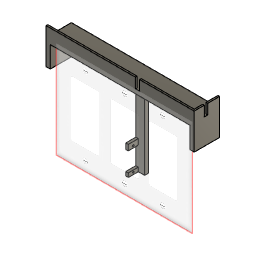
CPS_Project_Switch Mount v4 (Autodesk Fusion 360 design; units mm, degrees)
Autodesk Fusion 360 part; units mm, degrees
sketch "Sketch2" plane through (0, 0, 0) normal (0, 1, 0) x (1, 0, 0)
  line L0 (0, -62.2369) -> (87.5, -62.2369)
  line L1 (87.5, -62.2369) -> (87.5, -32.2369)
  line L2 (87.5, -32.2369) -> (82.5, -32.2369)
  line L3 (0, -57.2369) -> (0, -62.2369)
  line L4 (82.5, -32.2369) -> (82.5, -57.2369)
  line L5 (82.5, -57.2369) -> (0, -57.2369)
  line L6 (0, 0) -> (0, -57.2369) construction
  line L7 (-87.5, -32.2369) -> (-82.5, -32.2369)
  line L8 (-82.5, -32.2369) -> (-82.5, -57.2369)
  line L9 (-82.5, -57.2369) -> (0, -57.2369)
  line L10 (0, -57.2369) -> (0, -62.2369)
  line L11 (0, -62.2369) -> (-87.5, -62.2369)
  line L12 (-87.5, -62.2369) -> (-87.5, -32.2369)
  line L13 (0, 0) -> (30, 0) construction
  line L14 (0, 0) -> (0, -10.6) construction
  line L15 (18, 21.3) -> (28.4945, 21.3)
  line L16 (28.4945, 21.3) -> (28.4945, -57.2369)
  line L17 (28.4945, -57.2369) -> (18, -57.2369)
  line L18 (18, -57.2369) -> (18, 21.3)
  line L19 (21, -10.6) -> (18, -10.6)
  line L20 (18, -10.6) -> (18, -5.9)
  line L21 (18, -5.9) -> (21, -5.9)
  line L22 (21, -5.9) -> (21, -10.6)
  line L23 (0, 0) -> (0, 21.3) construction
  line L24 (18, 21.3) -> (21, 21.3)
  line L25 (21, 21.3) -> (21, 16.6)
  line L26 (21, 16.6) -> (18, 16.6)
  line L27 (18, 16.6) -> (18, 21.3)
  dimension "d1" = 5
  dimension "d2" = 82.5
  dimension "d3" = 5
  dimension "d4" = 25
  dimension "d10" = 10.6
  dimension "d14" = 4.7
  dimension "d15" = 3
  dimension "d16" = 21.3
  dimension "d17" = 3
  dimension "d18" = 4.7
  dimension "d19" = 22.5
  constraint horizontal L0
  constraint vertical L1
  constraint horizontal L2
  constraint vertical L3
  constraint vertical L4
  constraint horizontal L5
  constraint vertical L6
  constraint coincident L6.start L13.start
  constraint coincident L3.start L5.end
  constraint symmetric L0.start L6 L3.end
  constraint symmetric L0.end L6 L11.end
  constraint symmetric L1.end L6 L7.start
  constraint symmetric L2.end L6 L7.end
  constraint symmetric L4.end L6 L8.end
  constraint symmetric L3.start L6 L5.end
  constraint perpendicular L6 L13
  constraint horizontal L15
  constraint vertical L16
  constraint horizontal L17
  constraint vertical L18
  constraint coincident L5 L16.end
  constraint horizontal L19
  constraint vertical L20
  constraint horizontal L21
  constraint vertical L22
  constraint perpendicular L13 L23
  constraint horizontal L24
  constraint vertical L25
  constraint horizontal L26
  constraint vertical L27
  constraint coincident L18 L15.start
  constraint coincident L15.start L18.end
  measures "d1" distance of L1.end L2.end
  measures "d2" distance of L4.end L3.start
  measures "d3" distance of L0.start L3.start
  measures "d4" distance of L2.end L4.end
  measures "d10" distance of L6.start L14.end
  measures "d14" distance of L19.start L21.end
  measures "d15" distance of L19.start L19.end
  measures "d16" distance of L6.start L23.end
  measures "d17" distance of L15.start L24.end
  measures "d18" distance of L15.start L26.end
  measures "d19" distance of L20.end L26.end
extrude "Extrude1" add sketch "Sketch2" along normal blind 25 and the other way blind 5 contours L0 L1 L2 L3 L4 L5 L10 L17 | L3 L7 L8 L9 L10 L11 L12
extrude "Extrude2" add sketch "Sketch2" against normal blind 4.5 contours L5 L15 L16 L17 L18 L19 L21 L22 L25 L26 | L18 L19 L20 L21 L22 | L15 L18 L24 L25 L26 L27
extrude "Extrude3" add sketch "Sketch2" against normal blind 11.8 from surface at -4.5 contours L18 L19 L20 L21 L22 | L15 L18 L24 L25 L26 L27
sketch "Sketch3" plane through (21, 0, 0) normal (1, 0, 0) x (0, 1, 0)
  line L0 (-4.5, 5.9) -> (-4.5, 10.6)
  line L1 (-4.5, 10.6) -> (-16.3, 10.6)
  line L2 (-16.3, 10.6) -> (-16.3, 5.9)
  line L3 (-16.3, 5.9) -> (-4.5, 5.9)
  line L4 (-16.3, 10.6) -> (-10.4, 10.6) construction
  line L5 (-10.4, 10.6) -> (-10.4, 8.3) construction
  line L6 (-10.4, 8.3) -> (-16.3, 8.3) construction
  line L7 (-16.3, 8.3) -> (-16.3, 10.6) construction
  circle A0 centre (-10.4, 8.3) radius 1.1
  dimension "d23" = 5.9
  dimension "d24" = 2.3
  dimension "d25" = 2.2
  constraint horizontal L4
  constraint vertical L5
  constraint horizontal L6
  constraint vertical L7
  constraint coincident L1.end L2.start
  constraint coincident L5.end L6.start
  measures "d23" distance of L1.end L4.end
  measures "d24" distance of L1.end L6.end
  measures "d25" diameter of A0
sketch "Sketch4" plane through (21, 0, 0) normal (1, 0, 0) x (0, 1, 0)
  line L0 (-4.5, -21.3) -> (-4.5, -16.6)
  line L1 (-4.5, -16.6) -> (-16.3, -16.6)
  line L2 (-16.3, -16.6) -> (-16.3, -21.3)
  line L3 (-16.3, -21.3) -> (-4.5, -21.3)
  line L4 (-16.3, -16.6) -> (-10.4, -16.6) construction
  line L5 (-10.4, -16.6) -> (-10.4, -18.9) construction
  line L6 (-10.4, -18.9) -> (-16.3, -18.9) construction
  line L7 (-16.3, -18.9) -> (-16.3, -16.6) construction
  circle A0 centre (-10.4, -18.9) radius 1
  dimension "d26" = 5.9
  dimension "d27" = 2.3
  dimension "d28" = 2
  constraint horizontal L4
  constraint vertical L5
  constraint horizontal L6
  constraint vertical L7
  constraint coincident L1.end L2.start
  constraint coincident L5.end L6.start
  measures "d26" distance of L1.end L4.end
  measures "d27" distance of L1.end L6.end
  measures "d28" diameter of A0
extrude "Extrude4" cut sketch "Sketch4" against normal blind 6 contours A0
extrude "Extrude5" cut sketch "Sketch3" against normal blind 5.5 contours A0
extrude "Extrude6" add 1 faces at (20, -12.3667, 10.6) along direction (0, 0, 1) blind 2
sketch "Sketch5" plane through (0, 0, 62.2369) normal (0, 0, 1) x (-1, 0, 0)
  line L0 (-87.5, 5) -> (-87.5, -25)
  line L1 (-87.5, -25) -> (87.5, -25)
  line L2 (87.5, -25) -> (87.5, 5)
  line L3 (87.5, 5) -> (-87.5, 5)
  line L4 (87.5, 5) -> (-87.5, 5)
  line L5 (-87.5, 5) -> (-87.5, 3)
  line L6 (-87.5, 3) -> (87.5, 3)
  line L7 (87.5, 3) -> (87.5, 5)
  line L8 (-18.0867, 5) -> (-18.0867, 3)
  line L9 (-23.0002, 5) -> (-23.0002, 3)
  line L10 (-87.5, 3) -> (-85.5, 3)
  line L11 (-85.5, 3) -> (-85.5, -25)
  line L12 (-85.5, -25) -> (-87.5, -25)
  line L13 (-87.5, -25) -> (-87.5, 3)
  line L14 (-85.5, -11) -> (-87.5, -11)
  line L15 (-87.5, -11) -> (-87.5, -9)
  line L16 (-87.5, -9) -> (-85.5, -9)
  line L17 (-85.5, -9) -> (-85.5, -11)
  dimension "d35" = 2
  dimension "d38" = 2
  constraint horizontal L4
  constraint vertical L5
  constraint horizontal L6
  constraint vertical L7
  constraint coincident L2.end L3.start
  constraint coincident L3 L8.start
  constraint coincident L6 L8.end
  constraint perpendicular L6 L8
  constraint coincident L4 L9.start
  constraint coincident L6 L9.end
  constraint perpendicular L6 L9
  constraint horizontal L10
  constraint vertical L11
  constraint horizontal L12
  constraint vertical L13
  constraint horizontal L14
  constraint vertical L15
  constraint horizontal L16
  constraint vertical L17
  constraint coincident L13 L15.end
  constraint coincident L0 L15.end
  constraint midpoint L11 L14.start
  measures "d35" distance of L2.end L6.end
  measures "d38" distance of L5.end L10.end
extrude "Extrude7" add sketch "Sketch5" along normal blind 12 contours L0 L3 L4 L5 L6 L9 L10 | L2 L3 L4 L6 L7 L8
extrude "Extrude8" add sketch "Sketch5" along normal blind 12 contours L0 L6 L10 L11 L13 L16 | L0 L1 L11 L12 L13 L14
extrude "Extrude9" cut 1 faces at (86.8333, 9, 70.2369) along direction (0, -1, 0) blind 2
equation "d10 = 5.9 mm + 4.7 mm"
